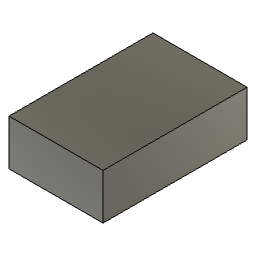
Container v4 (Autodesk Fusion 360 design; units mm, degrees)
Autodesk Fusion 360 part; units mm, degrees
sketch "Sketch1" plane through (0, 0, 0) normal (0, 0, 1) x (1, 0, 0)
  line L0 (0, 0) -> (98, 0)
  line L1 (98, 0) -> (98, 150)
  line L2 (98, 150) -> (0, 150)
  line L3 (0, 150) -> (0, 0)
  dimension "d1" = 98
  dimension "d2" = 150
  constraint horizontal L0
  constraint vertical L1
  constraint horizontal L2
  constraint vertical L3
  constraint coincident L0.start L3.end
  measures "d1" distance of L0.start L0.end
  measures "d2" distance of L0.start L2.end
extrude "Extrude1" add sketch "Sketch1" along normal blind 45
sketch "Sketch2" plane through (0, 0, 45) normal (0, 0, 1) x (-1, 0, 0)
  line L0 (0, -150) -> (0, 0)
  line L1 (0, 0) -> (-98, 0)
  line L2 (-98, 0) -> (-98, -150)
  line L3 (-98, -150) -> (0, -150)
  line L4 (0, 0) -> (-2.5, 0)
  line L5 (-2.5, 0) -> (-2.5, -2.5)
  line L6 (-2.5, -2.5) -> (-95.5, -2.5)
  line L7 (-95.5, -2.5) -> (-95.5, -147.5)
  line L8 (-95.5, -147.5) -> (-2.5, -147.5)
  line L9 (-2.5, -147.5) -> (-2.5, -2.5)
  dimension "d5" = 2.5
  dimension "d6" = 2.5
  dimension "d7" = 93
  dimension "d8" = 145
  constraint coincident L0.end L1.start
  constraint perpendicular L0 L4
  constraint perpendicular L1 L5
  constraint horizontal L6
  constraint vertical L7
  constraint horizontal L8
  constraint vertical L9
  measures "d5" distance of L0.end L4.end
  measures "d6" distance of L4.end L5.end
  measures "d7" distance of L5.end L6.end
  measures "d8" distance of L5.end L8.end
extrude "Extrude2" cut sketch "Sketch2" against normal blind 42.5 contours L6 L7 L8 L9
extrude "Extrude3" cut 1 faces at (2.5, 99.1667, 16.6667) along direction (-1, 0, 0) blind 2.5
sketch "Sketch3" plane through (95.5, 0, 0) normal (-1, 0, 0) x (0, -1, 0)
  line L0 (-2.5, 45) -> (-147.5, 45)
  line L1 (-147.5, 45) -> (-147.5, 2.5)
  line L2 (-147.5, 2.5) -> (-2.5, 2.5)
  line L3 (-2.5, 2.5) -> (-2.5, 45)
sketch "Sketch4" plane through (0, 147.5, 0) normal (0, -1, 0) x (1, 0, 0)
  line L0 (95.5, 45) -> (0, 45)
  line L1 (0, 45) -> (0, 2.5)
  line L2 (0, 2.5) -> (95.5, 2.5)
  line L3 (95.5, 2.5) -> (95.5, 45)
  line L4 (0, 0) -> (97.9689, 19.9489)
  constraint coincident L4.start origin
extrude "Extrude4" add sketch "Sketch4" along normal blind 145 contours L2 L3 L4
sketch "Sketch7" plane through (0, 0, 45) normal (0, 0, 1) x (-1, 0, 0)
  line L0 (0, -147.5) -> (-95.5, -147.5)
  line L1 (-95.5, -147.5) -> (-95.5, -2.5)
  line L2 (-95.5, -2.5) -> (0, -2.5)
  line L3 (0, -2.5) -> (0, 0)
  line L4 (0, 0) -> (-98, 0)
  line L5 (-98, 0) -> (-98, -150)
  line L6 (-98, -150) -> (0, -150)
  line L7 (0, -150) -> (0, -147.5)
  line L8 (-98, 0) -> (0, 0)
  line L9 (0, 0) -> (0, -150)
  line L10 (0, -150) -> (-98, -150)
  line L11 (-98, -150) -> (-98, 0)
  dimension "d19" = 98
  dimension "d20" = 150
  constraint horizontal L8
  constraint vertical L9
  constraint horizontal L10
  constraint vertical L11
  constraint coincident L4.end L5.start
  measures "d19" distance of L4.end L3.end
  measures "d20" distance of L4.end L5.end
extrude "Extrude5" add sketch "Sketch7" along normal blind 2.5
fillet "Fillet1" [suppressed]
fillet "Fillet2" [suppressed]
sketch "Sketch5" plane through (95.5, 0, 0) normal (-1, 0, 0) x (0, -1, 0)
sketch "Sketch6" plane through (95.5, 0, 0) normal (-1, 0, 0) x (0, -1, 0)
